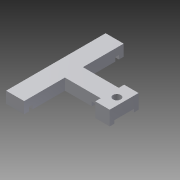
# Autodesk Inventor part: LongAxisTopClamp
Saved by Autodesk Inventor 2014 SP1 (Build 180222100, 222)
## iProperties
Created: 2017-05-20
Part Number: LongAxisTopClamp
Material: Generic
Document SubType Name: Modeling
Designer: danielsikar
Density: 1 g/cm^3
Appearance: White
Author: danielsikar
Autodesk Inventor part; units mm, degrees
ref_plane "Work Plane1" through (34.6017, 22.9, 27.7) normal (0, 0, 1) x (0, -1, 0)
sketch "Sketch1" plane through (34.6017, 22.9, 27.7) normal (0, 0, 1) x (0, -1, 0)
  line L0 (-22.65, -5.5017) -> (22.65, -5.5017)
  line L1 (22.65, -5.5017) -> (22.65, -15.5017)
  line L2 (22.65, -15.5017) -> (-22.65, -15.5017)
  line L3 (-22.65, -15.5017) -> (-22.65, -5.5017)
  line L4 (-23.05, -33.7017) -> (-23.05, 15.1916) construction
  line L5 (23.05, 15.1916) -> (23.05, -33.7017) construction
  line L6 (-23.95, -33.6017) -> (-23.95, 15.3983) construction
  line L7 (22.9493, -34.6017) -> (-22.9493, -34.6017) construction
  line L8 (-23.85, -35.5017) -> (23.85, -35.5017) construction
  line L9 (23.05, -33.7017) -> (-23.05, -33.7017) construction
  point P0 (22.9, -34.6017)
  dimension "d0" = 45.3
  dimension "d1" = 10
  dimension "d2" = 0.4
  dimension "d4" = 20
  constraints: 8 end point, 2 parallel, 1 horizontal, 1 perpendicular
  measures "d0" distance of L1.end L2.end
  measures "d1" distance of L0.end L1.end
  measures "d2" distance between parallel lines of L5 L1
  measures "d4" distance between parallel lines of L8 L2
extrude "Extrusion1" add sketch "Sketch1" along normal blind 3
sketch "Sketch2" plane through (19.1, 45.55, 27.7) normal (0, 1, 0) x (1, 0, 0)
  line L0 (10, 0) -> (10, -3) projected
  line L1 (0, -3) -> (10, -3)
  line L2 (10, -3) -> (10, -0.9)
  line L3 (10, -0.9) -> (0, -0.9)
  line L4 (0, -0.9) -> (0, -3)
  point P0 (-19.1, 27.7)
  dimension "d7" = 2.1
  constraints: 8 end point, 2 parallel, 1 horizontal, 1 perpendicular, 1 point on line
  measures "d7" distance of L2.end L1.end
extrude "Extrusion2" add sketch "Sketch2" along normal blind 2
ref_plane "Work Plane3" through (19.1, 22.9, 27.7) normal (0, -1, 0) x (1, 0, 0)
mirror "Mirror2" about plane through (19.1, 22.9, 27.7) normal (0, -1, 0) of "Extrusion2"
sketch "Sketch3" plane through (19.1, 0.25, 27.7) normal (0, -1, 0) x (1, 0, 0)
  line L0 (10, 0.9) -> (0, 0.9) projected
  line L1 (0, 0) -> (0, 0.9) projected
  line L2 (10, 0) -> (0, 0) projected
  line L3 (10, 0) -> (10, 0.9) projected
  point P0 (-19.1, -27.7)
extrude "Extrusion3" add sketch "Sketch3" along normal blind 0.2
sketch "Sketch4" plane through (19.1, 45.55, 27.7) normal (0, 1, 0) x (1, 0, 0)
  line L0 (0, -0.9) -> (10, -0.9) projected
  line L1 (10, 0) -> (10, -0.9) projected
  line L2 (0, 0) -> (10, 0) projected
  line L3 (0, 0) -> (0, -0.9) projected
  point P0 (-19.1, 27.7)
extrude "Extrusion4" add sketch "Sketch4" along normal blind 0.2
sketch "Sketch5" plane through (19.1, 47.55, 27.7) normal (0, 1, 0) x (1, 0, 0)
  line L0 (0, -3) -> (10, -3) projected
  line L1 (10, -3) -> (10, -0.9) projected
  line L2 (10, -0.9) -> (0, -0.9) projected
  line L3 (0, -0.9) -> (0, -3) projected
  point P0 (-19.1, 27.7)
extrude "Extrusion5" add sketch "Sketch5" along normal blind 1.6
sketch "Sketch6" plane through (19.1, -1.75, 30.7) normal (0, -1, 0) x (1, 0, 0)
  line L0 (0, 0) -> (10, 0) projected
  line L1 (0, -2.1) -> (0, 0) projected
  line L2 (10, -2.1) -> (0, -2.1) projected
  line L3 (10, 0) -> (10, -2.1) projected
  point P0 (-19.1, -30.7)
extrude "Extrusion6" add sketch "Sketch6" along normal blind 1.6
sketch "Sketch7" plane through (29.1, 45.75, 28.6) normal (0, 0, -1) x (-1, 0, 0)
  line L0 (10, 0) -> (10, 3.4) projected
  line L1 (0, 3.4) -> (10, 3.4)
  line L2 (10, 3.4) -> (10, 1.85)
  line L3 (10, 1.85) -> (0, 1.85)
  line L4 (0, 1.85) -> (0, 3.4)
  point P0 (29.1, -45.75)
  dimension "d20" = 1.55
  constraints: 8 end point, 2 parallel, 1 horizontal, 1 perpendicular, 1 point on line
  measures "d20" distance of L1.end L2.end
extrude "Extrusion7" add sketch "Sketch7" along normal up to surface (0.9 mm away)
mirror "Mirror3" about plane through (19.1, 22.9, 27.7) normal (0, -1, 0) of "Extrusion7"
sketch "Sketch8" plane through (19.1, 47.6, 28.6) normal (0, -1, 0) x (1, 0, 0)
  line L0 (0, -0.9) -> (10, -0.9) projected
  line L1 (10, 0) -> (10, -0.9) projected
  line L2 (0, 0) -> (10, 0) projected
  line L3 (0, 0) -> (0, -0.9) projected
  point P0 (-19.1, -28.6)
extrude "Extrusion8" cut sketch "Sketch8" against normal blind 0.2
sketch "Sketch9" plane through (19.1, -1.8, 27.7) normal (0, 1, 0) x (1, 0, 0)
  line L0 (0, 0) -> (10, 0) projected
  line L1 (0, -0.9) -> (0, 0) projected
  line L2 (10, -0.9) -> (0, -0.9) projected
  line L3 (10, -0.9) -> (10, 0) projected
  point P0 (-19.1, 27.7)
extrude "Extrusion9" cut sketch "Sketch9" against normal blind 0.2
sketch "Sketch10" plane through (34.6017, 22.9, 30.7) normal (0, 0, 1) x (1, 0, 0)
  line L0 (-5.5017, 26.25) -> (-5.5017, -26.25) projected
  line L1 (-15.5017, 26.25) -> (-5.5017, 26.25) projected
  line L2 (-15.5017, -26.25) -> (-15.5017, 26.25) projected
  line L3 (-5.5017, -26.25) -> (-15.5017, -26.25) projected
  point P0 (-34.6017, -22.9)
extrude "Extrusion10" add sketch "Sketch10" along normal blind 2
sketch "Sketch11" plane through (29.1, 0.05, 27.7) normal (1, 0, 0) x (0, 0, -1)
  line L0 (0, 45.7) -> (0, 0) projected
  line L1 (-5, -3.4) -> (-5, 49.1) projected
  line L2 (-5, 27.85) -> (0, 27.85)
  line L3 (0, 27.85) -> (0, 17.85)
  line L4 (0, 17.85) -> (-5, 17.85)
  line L5 (-5, 17.85) -> (-5, 27.85)
  line L6 (0, 49.1) -> (-5, 49.1) projected
  point P0 (27.7, -0.05)
  dimension "d29" = 10
  dimension "d37" = 21.25
  constraints: 8 end point, 2 parallel, 2 point on line, 1 horizontal, 1 perpendicular
  measures "d29" distance of L2.end L3.end
  measures "d37" distance between parallel lines of L2 L6
ref_plane "Work Plane4" through (53.9, 4.4, -9.45) normal (1, 0, 0) x (0, 1, 0)
ref_plane "Work Plane5" through (56.9, 17.9, 20.2) normal (1, 0, 0) x (0, 1, 0)
extrude "Extrusion11" add sketch "Sketch11" along normal up to surface (27.8 mm away)
sketch "Sketch12" plane through (29.1, 17.9, 27.7) normal (0, -1, 0) x (1, 0, 0)
  line L0 (16.8, 0) -> (16.8, 0.8) construction
  line L1 (15.8, 0.8) -> (16.8, 0.8) construction
  line L2 (15, 0) -> (15, 0.8) construction
  line L3 (27.8, 0) -> (27.8, 5) construction
  line L4 (0, 5) -> (27.8, 5) construction
  line L5 (0, 0) -> (0, 5) construction
  line L6 (0, 0) -> (27.8, 0) construction
  line L7 (-34.3067, 0.8) -> (15.8, 0.8) construction
  line L8 (15, 0) -> (15, 0.8) construction
  line L9 (15, 0) -> (15, 0.8)
  line L10 (16.8, 0.8) -> (16.8, 0)
  line L11 (15, 0) -> (16.8, 0)
  line L12 (16.8, 0) -> (16.8, 0.8)
  line L13 (16.8, 0.8) -> (15, 0.8)
  line L14 (15, 0.8) -> (15, 0)
  line L15 (14.9, 0) -> (16.9, 0)
  line L16 (16.9, 0) -> (16.9, 1)
  line L17 (16.9, 1) -> (14.9, 1)
  line L18 (14.9, 1) -> (14.9, 0)
  point P0 (-29.1, -27.7)
  dimension "d32" = 2
  dimension "d33" = 1
  dimension "d34" = 0.1
  constraints: 22 end point, 6 equal length, 3 perpendicular, 2 horizontal, 1 point on line
  measures "d32" distance of L17.end L16.end
  measures "d33" distance of L16.end L15.end
  measures "d34" distance between parallel lines of L18 L2
extrude "Extrusion12" cut sketch "Sketch12" against normal up to next
sketch "Sketch17" plane through (34.6017, 22.9, 32.7) normal (0, 0, 1) x (1, 0, 0)
  circle A0 centre (18.2983, 0) radius 2.15 projected
  point P0 (-34.6017, -22.9)
extrude "Extrusion16" cut sketch "Sketch17" against normal up to next
sketch "Sketch18" plane through (56.9, 17.9, 27.7) normal (1, 0, 0) x (0, 0, -1)
  line L0 (0, 0) -> (-5, 0) projected
  line L1 (0, 10) -> (0, 0) projected
  line L2 (-5, 10) -> (0, 10) projected
  line L3 (-5, 0) -> (-5, 10) projected
  point P0 (27.7, -17.9)
extrude "Extrusion17" add sketch "Sketch18" along normal blind 3
sketch "Sketch20" plane through (29.1, 17.9, 27.7) normal (0, -1, 0) x (1, 0, 0)
  line L0 (16.9, 0) -> (30.8, 0) projected
  line L1 (30.8, 5) -> (19.8, 5)
  line L2 (19.8, 5) -> (19.8, 0)
  line L3 (19.8, 0) -> (30.8, 0)
  line L4 (30.8, 0) -> (30.8, 5)
  point P0 (-29.1, -27.7)
  dimension "d51" = 11
  constraints: 8 end point, 2 parallel, 1 horizontal, 1 perpendicular, 1 point on line
  measures "d51" distance of L3.end L2.end
extrude "Extrusion18" add sketch "Sketch20" along normal blind 3
sketch "Sketch21" plane through (29.1, 27.9, 32.7) normal (0, 1, 0) x (1, 0, 0)
  line L0 (16.9, 5) -> (30.8, 5) projected
  line L1 (30.8, 0) -> (19.8, 0)
  line L2 (19.8, 0) -> (19.8, 5)
  line L3 (19.8, 5) -> (30.8, 5)
  line L4 (30.8, 5) -> (30.8, 0)
  point P0 (-29.1, 32.7)
  dimension "d54" = 11
  constraints: 8 end point, 2 parallel, 1 horizontal, 1 perpendicular, 1 point on line
  measures "d54" distance of L2.end L3.end
extrude "Extrusion19" add sketch "Sketch21" along normal blind 3
sketch "Sketch22" plane through (34.6017, 22.9, 27.7) normal (0, 0, -1) x (-1, 0, 0)
  line L0 (-14.2983, -8) -> (-22.2983, -8)
  line L1 (-22.2983, -8) -> (-22.2983, -5.5)
  line L2 (-22.2983, -5.5) -> (-14.2983, -5.5)
  line L3 (-14.2983, -5.5) -> (-14.2983, -8)
  point P0 (34.6017, -22.9)
  dimension "d57" = 8
  dimension "d58" = 2.5
  constraints: 8 end point, 2 parallel, 1 horizontal, 1 perpendicular
  measures "d57" distance of L1.end L2.end
  measures "d58" distance of L0.end L1.end
extrude "Extrusion20" add sketch "Sketch22" along normal blind 3
sketch "Sketch23" plane through (34.6017, 22.9, 27.7) normal (0, 0, -1) x (-1, 0, 0)
  line L0 (-14.2983, 8) -> (-22.2983, 8)
  line L1 (-22.2983, 8) -> (-22.2983, 5.5)
  line L2 (-22.2983, 5.5) -> (-14.2983, 5.5)
  line L3 (-14.2983, 5.5) -> (-14.2983, 8)
  point P0 (34.6017, -22.9)
  dimension "d61" = 8
  dimension "d62" = 2.5
  constraints: 8 end point, 2 parallel, 1 horizontal, 1 perpendicular
  measures "d61" distance of L2.end L1.end
  measures "d62" distance of L1.end L0.end
extrude "Extrusion21" add sketch "Sketch23" along normal blind 3
sketch "Sketch24" plane through (59.9, 17.9, 27.7) normal (1, 0, 0) x (0, 0, -1)
  line L0 (0, 13) -> (0, -3) projected
  line L1 (-5, 13) -> (0, 13) projected
  line L2 (-5, -3) -> (-5, 13) projected
  line L3 (0, -3) -> (-5, -3) projected
  point P0 (27.7, -17.9)
extrude "Extrusion22" cut sketch "Sketch24" against normal blind 3
sketch "Sketch25" plane through (34.6017, 22.9, 27.7) normal (0, 0, -1) x (-1, 0, 0)
  line L0 (-9.3983, 5) -> (-9.3983, -5) projected
  line L1 (5.5017, -5) -> (-9.3983, -5) projected
  line L2 (5.5017, -5) -> (5.5017, -22.85) projected
  line L3 (15.5017, -22.85) -> (5.5017, -22.85) projected
  line L4 (15.5017, -22.85) -> (15.5017, 22.85) projected
  line L5 (5.5017, 22.85) -> (15.5017, 22.85) projected
  line L6 (5.5017, 22.85) -> (5.5017, 5) projected
  line L7 (5.5017, 5) -> (-9.3983, 5) projected
  point P0 (34.6017, -22.9)
extrude "Extrusion23" add sketch "Sketch25" along normal blind 1.3
sketch "Sketch26" plane through (19.1, -3.35, 30.7) normal (0, -1, 0) x (1, 0, 0)
  line L0 (0, -3) -> (0, 2) projected
  line L1 (10, -3) -> (0, -3) projected
  line L2 (10, 2) -> (10, -3) projected
  line L3 (0, 2) -> (10, 2) projected
  point P0 (-19.1, -30.7)
extrude "Extrusion24" add sketch "Sketch26" along normal blind 1.3
sketch "Sketch27" plane through (19.1, 49.15, 27.7) normal (0, 1, 0) x (1, 0, 0)
  line L0 (10, 0) -> (10, -5) projected
  line L1 (10, 0) -> (0, 0) projected
  line L2 (0, -5) -> (0, 0) projected
  line L3 (10, -5) -> (0, -5) projected
  point P0 (-19.1, 27.7)
extrude "Extrusion25" add sketch "Sketch27" along normal blind 1.3
sketch "Sketch28" plane through (29.1, 47.8, 27.7) normal (0, 0, -1) x (-1, 0, 0)
  line L0 (0, 0) -> (10, 0) projected
  line L1 (10, 0) -> (10, 2.65) projected
  line L2 (0, 2.65) -> (10, 2.65) projected
  line L3 (0, 0) -> (0, 2.65) projected
  point P0 (29.1, -47.8)
extrude "Extrusion26" add sketch "Sketch28" along normal blind 1.3
sketch "Sketch29" plane through (29.1, -2, 27.7) normal (0, 0, -1) x (-1, 0, 0)
  line L0 (10, 0) -> (0, 0) projected
  line L1 (0, 0) -> (0, -2.65) projected
  line L2 (10, -2.65) -> (0, -2.65) projected
  line L3 (10, -2.65) -> (10, 0) projected
  point P0 (29.1, 2)
extrude "Extrusion27" add sketch "Sketch29" along normal blind 1.3
sketch "Sketch30" plane through (34.6017, 22.9, 27.7) normal (0, 0, -1) x (-1, 0, 0)
  circle A0 centre (-18.2983, 0) radius 2.15 projected
  line L0 (-22.2983, 5.5) -> (-22.2983, -5.5) projected
  line L1 (-22.2983, -5.5) -> (-14.2983, -5.5) projected
  line L2 (-14.2983, -5) -> (-14.2983, -5.5) projected
  line L3 (-11.3983, -5) -> (-14.2983, -5) projected
  line L4 (-11.3983, -5) -> (-11.3983, 5) projected
  line L5 (-11.3983, 5) -> (-14.2983, 5) projected
  line L6 (-14.2983, 5) -> (-14.2983, 5.5) projected
  line L7 (-14.2983, 5.5) -> (-22.2983, 5.5) projected
  point P0 (34.6017, -22.9)
extrude "Extrusion28" add sketch "Sketch30" along normal blind 1.3
body "Solid1"
